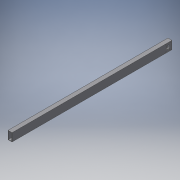
# Autodesk Inventor part: 34.48in Arm Bea
Saved by Autodesk Inventor 2018 (Build 220112000, 112)
## iProperties
Created: 2019-01-17
Part Number: 34.48in Arm Bea
Material: Generic
Document SubType Name: Modeling
Designer: Gabriel
Density: 1 g/cm^3
Appearance: Default
Author: Gabriel
Autodesk Inventor part; units mm, degrees
ref_plane "YZ Plane" through (0, 0, 0) normal (1, 0, 0) x (0, 1, 0)
ref_plane "XZ Plane" through (0, 0, 0) normal (0, 1, 0) x (-1, 0, 0)
ref_plane "XY Plane" through (0, 0, 0) normal (0, 0, 1) x (1, 0, 0)
sketch "Sketch1" plane through (0, 0, 0) normal (0, 0, 1) x (1, 0, 0)
  line L0 (-35.3228, 16.049) -> (-9.9228, 16.049)
  line L1 (-9.9228, 16.049) -> (-9.9228, -34.751)
  line L2 (-9.9228, -34.751) -> (-35.3228, -34.751)
  line L3 (-35.3228, -34.751) -> (-35.3228, 16.049)
  line L4 (-13.0978, 12.874) -> (-32.1478, 12.874)
  line L5 (-32.1478, 12.874) -> (-32.1478, -31.576)
  line L6 (-32.1478, -31.576) -> (-13.0978, -31.576)
  line L7 (-13.0978, -31.576) -> (-13.0978, 12.874)
  point P0 (0, 0)
  dimension "d0" = 25.4
  dimension "d1" = 50.8
  dimension "d2" = 3.175
  constraints: 16 end point, 4 parallel, 2 perpendicular, 1 horizontal, 3 other
  measures "d0" distance of L1.end L2.end
  measures "d1" distance of L0.end L1.end
  measures "d2" distance between parallel lines of L0 L4
extrude "Extrusion1" add sketch "Sketch1" along normal blind 1008.38
sketch "Sketch2" plane through (-35.3228, -34.751, 0) normal (-1, 0, 0) x (0, 0, 1)
  line L0 (0, 0) -> (0, 50.8) construction
  line L1 (0, 25.4) -> (25.4, 25.4) construction
  circle A0 centre (25.4, 25.4) radius 12.7
  point P0 (0, 34.751)
  dimension "d5" = 25.4
  dimension "d9" = 25.4
  constraints: 2 end point, 1 centre point, 1 coincident, 1 horizontal, 1 midpoint
  measures "d5" distance of L1.start L1.end
  measures "d9" diameter of A0
extrude "Extrusion2" cut sketch "Sketch2" against normal blind 254
sketch "Sketch3" plane through (-35.3228, -34.751, 0) normal (-1, 0, 0) x (0, 0, 1)
  line L0 (0, 50.8) -> (1008.38, 50.8) construction
  line L1 (0, 50.8) -> (0, 46.0248) construction
  line L2 (0, 0) -> (0, 50.8) construction
  line L3 (0, 46.0248) -> (13.4874, 46.0248) construction
  line L4 (13.4874, 46.0248) -> (37.3126, 46.0248) construction
  line L5 (13.4874, 46.0248) -> (13.4874, 4.7752) construction
  line L6 (37.3126, 46.0248) -> (37.3126, 4.7752) construction
  circle A0 centre (13.4874, 4.7752) radius 2.5797
  circle A1 centre (37.3126, 4.7752) radius 2.5797
  circle A2 centre (37.3126, 46.0248) radius 2.5797
  circle A3 centre (13.4874, 46.0248) radius 2.5797
  point P0 (0, 34.751)
  dimension "d10" = 4.7752
  dimension "d11" = 13.4874
  dimension "d12" = 23.8252
  dimension "d13" = 41.2496
  dimension "d14" = 41.2496
  dimension "d15" = 5.1594
  dimension "d16" = 5.1594
  dimension "d17" = 5.1594
  dimension "d18" = 5.1594
  constraints: 10 end point, 4 centre point, 4 coincident, 2 point on line, 2 vertical, 1 perpendicular
  measures "d10" distance of L0.start L1.end
  measures "d11" distance of L1.end L3.end
  measures "d12" distance of L3.end L4.end
  measures "d13" distance of L3.end L5.end
  measures "d14" distance of L4.end L6.end
  measures "d15" diameter of A0
  measures "d16" diameter of A1
  measures "d17" diameter of A2
  measures "d18" diameter of A3
extrude "Extrusion3" cut sketch "Sketch3" against normal blind 25.4
body "Solid1"
